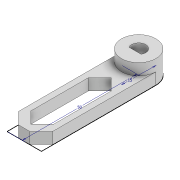
# Autodesk Inventor part: StepMotorTest
Saved by Autodesk Inventor 2020.3 (Build 243373000, 373)
## iProperties
Created: 2021-05-24
Part Number: StepMotorTest
Material: Generic
Document SubType Name: Modeling
Designer: Yusuf
Mass: 3.20638 g
Surface Area: 24.5195 cm^2
Volume: 3.20638 cm^3
Density: 1 g/cm^3
Appearance: Default
Author: Yusuf
Autodesk Inventor part; units mm, degrees
ref_plane "YZ Plane" through (0, 0, 0) normal (1, 0, 0) x (0, 1, 0)
ref_plane "XZ Plane" through (0, 0, 0) normal (0, 1, 0) x (-1, 0, 0)
ref_plane "XY Plane" through (0, 0, 0) normal (0, 0, 1) x (1, 0, 0)
sketch "Sketch1" plane through (0, 0, 0) normal (0, 1, 0) x (-1, 0, 0)
  arc A0 (-2.2913, 1) -> (2.2913, 1) centre (0, 0) ccw
  circle A1 centre (0, 0) radius 3.088
  line L0 (2.6552, 1.6) -> (-2.6552, 1.6)
  line L1 (-2.6411, 1.6) -> (2.6552, 1.6)
  line L2 (2.2913, 1) -> (-2.2913, 1)
  circle A2 centre (0, 0) radius 7.5
  line L3 (7.5, 0) -> (7.5, 50)
  line L4 (7.5, 50) -> (-7.5, 50)
  line L5 (-7.5, 50) -> (-7.5, 0)
  point P0 (2.6411, 1.6)
  point P1 (-2.6411, 1.6)
  dimension "d1" = 15
  dimension "d2" = 50
  constraints: 12 end point, 4 point on circle, 2 centre point, 2 coincident, 1 collinear, 1 parallel, 1 perpendicular, 1 tangent, 1 vertical, 3 other
  measures "d1" diameter of A2
  measures "d2" distance of L3.start L3.end
extrude "Extrusion1" add sketch "Sketch1" along normal blind 10 contours A1 L0 | A2 picked at (0.7371, 1.7852)
extrude "Extrusion2" add sketch "Sketch1" along normal blind 5 contours A2 L5 L4 L3
chamfer "Chamfer1" distance 5 angle 45 2 edges at (-7.5, 2.5, 50) (7.5, 2.5, 50)
sketch "Sketch3" plane through (0, 0, 0) normal (0, -1, 0) x (1, 0, 0)
  line L0 (-5, 42) -> (0, 47)
  line L1 (-2.5, 50) -> (-7.5, 45) projected
  line L2 (0, 47) -> (5, 42)
  line L3 (5, 42) -> (-5, 42)
  line L4 (-5, 42) -> (-5, 12)
  line L5 (5, 12) -> (5, 42)
  line L6 (-2.5, 50) -> (2.5, 50) projected
  line L7 (-5, 12) -> (-5, 5.5902)
  arc A0 (7.5, 0) -> (-7.5, 0) centre (0, 0) ccw projected
  line L8 (5, 12) -> (5, 5.5902)
  circle A1 centre (0, 0) radius 7.5 projected
  line L9 (5, 12) -> (-5, 12)
  dimension "d13" = 10
  dimension "d14" = 30
  dimension "d15" = 3
  constraints: 16 end point, 3 vertical, 2 perpendicular, 2 point on circle, 1 horizontal, 1 parallel
  measures "d13" distance between parallel lines of L4 L5
  measures "d14" distance of L5.start L2.end
  measures "d15" distance from line of L6 L0.end
extrude "Extrusion3" cut sketch "Sketch3" against normal blind 5.5 contours L0 L2 L3 | L3 L5 L9 L4
chamfer "Chamfer2" distance 5 angle 45 2 edges at (-5, 2.5, 12) (5, 2.5, 12)
body "Solid1"
